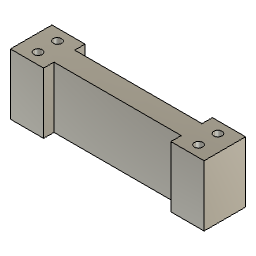
smart-grind-by-weight. Eureka Mignon (Autodesk Fusion 360 archive; units mm, degrees)
design "Load cell"
Autodesk Fusion 360 part; units mm, degrees
sketch "Sketch3" plane through (0, 0, 0) normal (0, 0, 1) x (1, 0, 0)
  line L0 (-35, 0) -> (35, 0) construction
  line L1 (-35, 7.5) -> (-35, -7.5)
  line L2 (35, 7.5) -> (35, -7.5)
  line L3 (-23, -3.75) -> (23, -3.75)
  line L4 (-23, 3.75) -> (23, 3.75)
  line L5 (0, 3.75) -> (0, -3.75) construction
  line L6 (-35, -7.5) -> (-23, -7.5)
  line L7 (35, -7.5) -> (23, -7.5)
  line L8 (-35, 7.5) -> (-23, 7.5)
  line L9 (-23, 3.75) -> (23, 3.75)
  line L10 (35, 7.5) -> (23, 7.5)
  circle A0 centre (-29, 3.5) radius 1.5
  circle A1 centre (-29, -3.5) radius 1.5
  circle A2 centre (29, 3.5) radius 1.5
  circle A3 centre (29, -3.5) radius 1.5
  line L11 (-29, 3.5) -> (-29, -3.5) construction
  line L12 (29, 3.5) -> (29, -3.5) construction
  line L13 (29, -3.5) -> (-29, -3.5) construction
  line L14 (-29, -3.5) -> (29, 3.5) construction
  line L15 (23, -7.5) -> (23, -3.75)
  line L16 (23, 3.75) -> (23, 7.5)
  line L17 (-23, 7.5) -> (-23, 3.75)
  line L18 (-23, -7.5) -> (-23, -3.75)
  dimension "d9" = 70
  dimension "d10" = 15
  dimension "d13" = 7.5
  dimension "d17" = 3
  dimension "d18" = 3
  dimension "d19" = 3
  dimension "d20" = 3
  dimension "d22" = 7
  dimension "d23" = 7
  dimension "d26" = 6
  dimension "d27" = 12
  constraint horizontal L0
  constraint midpoint origin L0
  constraint vertical L1
  constraint midpoint L0.start L1
  constraint perpendicular L0 L2
  constraint equal L1 L2
  constraint midpoint L0.end L2
  constraint horizontal L3
  constraint horizontal L4
  constraint equal L3 L4
  constraint midpoint L4 L5.start
  constraint midpoint L3 L5.end
  constraint midpoint origin L5
  constraint perpendicular L1 L6
  constraint vertical L5
  constraint perpendicular L2 L7
  constraint symmetric L0 L1.end L1.start
  constraint symmetric L0 L2.end L2.start
  constraint symmetric L0 L3.start L4.start
  constraint symmetric L0 L3.end L4.end
  constraint symmetric L0 L6.end L8.end
  constraint symmetric L0 L7.end L10.end
  constraint coincident A0.centre L11.start
  constraint coincident A1.centre L11.end
  constraint vertical L11
  constraint coincident A3.centre L12.end
  constraint vertical L12
  constraint horizontal L13
  constraint coincident A2.centre L12.start
  constraint midpoint origin L14
  constraint parallel L15 L17
  constraint vertical L17
  measures "d9" distance of L0.start L0.end
  measures "d10" distance of L1.start L1.end
  measures "d13" distance of L3 L4
  measures "d17" diameter of A0
  measures "d18" diameter of A1
  measures "d19" diameter of A2
  measures "d20" diameter of A3
  measures "d22" vertical distance of A0.centre A1.centre
  measures "d23" vertical distance of A2.centre A3.centre
  measures "d26" distance of L1 A0.centre
  measures "d27" distance of L10.end L2.start
extrude "Extrude2" add sketch "Sketch3" along normal blind 22

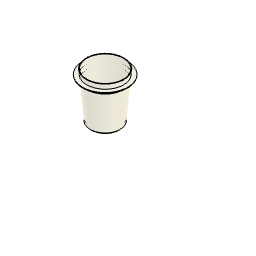
design "Dosing cup"
Autodesk Fusion 360 part; units mm, degrees
ref_plane "WorkPlane1" through (0, -100.5, 0) normal (0, 1, 0) x (0, 0, 1)
sketch "Sketch2" plane through (0, -100.5, 0) normal (0, 1, 0) x (1, 0, 0)
  line L0 (-20, -66.2) -> (20, -66.2)
  line L1 (-20, -66.2) -> (20, -66.2)
  line L2 (-22, -68.2) -> (22, -68.2) construction
  line L3 (11.75, -145.6805) -> (-11.75, -145.6805)
  line L4 (0, -134.97) -> (0, -66.2)
  line L5 (0, -66.2) -> (19.7, -66.2)
  line L6 (21.9996, -68.5) -> (27.75, -134.97)
  line L7 (27.75, -134.97) -> (0, -134.97)
  line L8 (20, -66.2) -> (22, -66.2) construction
  line L9 (22, -66.2) -> (22, -68.2) construction
  arc A0 (19.7, -66.2) -> (21.9996, -68.5) centre (22, -66.2) ccw
  line L10 (21.265, -71.6106) -> (27.5184, -143.8956)
  line L11 (1, -67.2) -> (16.6321, -67.2)
  arc A1 (16.6321, -67.2) -> (21.265, -71.6106) centre (22, -66.2) ccw
  line L12 (27.5184, -143.8956) -> (26.7463, -134.97)
  line L13 (1, -67.2) -> (0, -67.2)
  line L14 (27.145, -127.9772) -> (33.1445, -127.8996)
  line L15 (33.1445, -127.8996) -> (33.1316, -126.8997)
  line L16 (33.1316, -126.8997) -> (27.0586, -126.9782)
  line L17 (-4.1, -71) -> (4.1, -71)
  line L18 (4.1, -71) -> (4.1, -66.2)
  line L19 (4.1, -66.2) -> (-4.1, -66.2)
  line L20 (-4.1, -66.2) -> (-4.1, -71)
  line L21 (0, -72) -> (21.2986, -72)
  line L22 (33.1316, -126.8997) -> (32.8451, -126.9034)
  line L23 (33.1316, -126.8997) -> (42.5674, -126.8997) construction
  line L24 (33.1316, -126.8997) -> (26.5749, -121.3872)
  line L25 (-20, -66.2) -> (20, -66.2)
  point P0 (0, -71)
  dimension "d251" = 27.75
  dimension "d252" = 0.3
  dimension "d253" = 0.3
  dimension "d255" = 6
  dimension "d256" = 7
  dimension "d257" = 1
  dimension "d258" = 8.2
  dimension "d259" = 4.8
  dimension "d260" = 1
  dimension "d263" = 45
  dimension "d264" = 68.77
  constraint midpoint L1 L4.end
  constraint perpendicular L4 L5
  constraint parallel L2 L7
  constraint coincident L1 L5.end
  constraint coincident L0.end L1.end
  constraint parallel L1 L8
  constraint coincident L2.end L9.end
  constraint coincident L8.end L9.start
  constraint coincident L7 L12.end
  constraint parallel L10 L12
  constraint coincident L4 L13.end
  constraint perpendicular L4 L13
  constraint coincident L6 L14.start
  constraint perpendicular L14 L15
  constraint coincident L6 L16.end
  constraint perpendicular L15 L16
  constraint concentric A0 A1
  constraint horizontal L17
  constraint vertical L18
  constraint horizontal L19
  constraint vertical L20
  constraint collinear L5 L19
  constraint midpoint L17 P0
  constraint coincident L4 P0
  constraint coincident L4 L21.start
  constraint coincident L10 L21.end
  constraint perpendicular L4 L21
  constraint coincident L16 L22.end
  constraint perpendicular L15 L22
  constraint horizontal L23
  constraint coincident L6 L24.end
  measures "d251" distance of L4.start L6.end
  measures "d252" distance of L0.end L5.end
  measures "d253" distance of L2.end L6.start
  measures "d255" distance of L14.start L14.end
  measures "d256" distance of L6.end L14
  measures "d257" distance of L14.end L15.end
  measures "d258" distance of L17.start L17.end
  measures "d259" distance of L17.start L19.end
  measures "d260" distance of L17 L21
  measures "d263" angle of L6 L24
  measures "d264" distance of L7 L25
revolve "Revolve1" add sketch "Sketch2" angle 360 about axis through (0, -100.5, 134.97) along (0, 0, -1) contours L0 L1 L5 L6 L7 A0 L10 L11 A1 L18 L25 | L4 L10 L11 A1 L17 L18 L21 | L6 L16 L22 L24 | L6 L14 L15 L16 L22
equation "d251 = ( 55.5 / 2 ) * 1 mm"
named bodies: "dosing cup"
